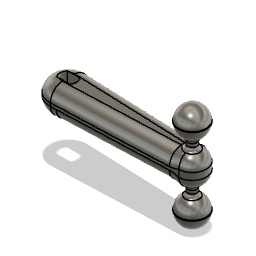
bicep (Autodesk Fusion 360 design; units mm, degrees)
Autodesk Fusion 360 part; units mm, degrees
sketch "Sketch1" plane through (0, 0, 0) normal (0, 1, 0) x (1, 0, 0)
  circle A0 centre (0, 0) radius 2.7
  line L0 (-2.056089, 1.75) -> (2.056089, 1.75)
  line L1 (-2.137171, -1.65) -> (2.137171, -1.65)
  circle A1 centre (0, 0) radius 6
  circle A2 centre (40, 0) radius 4.5
  line L2 (40.16875, 4.496835) -> (0.225, 5.99578)
  line L3 (0.225, -5.99578) -> (40.16875, -4.496835)
  circle A3 centre (40, 0) radius 1.5
  dimension "d1" = 5.4
  dimension "d2" = 3.4
  dimension "d3" = 1.75
  dimension "d4" = 12
  dimension "d10" = 9
  dimension "d11" = 40
  dimension "d14" = 3
  constraint coincident A0.centre A1.centre
  constraint horizontal L0
  constraint parallel L0 L1
  constraint concentric A0 A1
  constraint tangent A1 L2
  constraint tangent A2 L3
  constraint horizontal A0.centre A2.centre
  constraint tangent A1 L3
  constraint tangent A2 L2
  constraint concentric A2 A3
  measures "d1" diameter of A0
  measures "d2" distance of L0 L1
  measures "d3" distance of A0.centre L0
  measures "d4" diameter of A1
  measures "d10" diameter of A2
  measures "d11" distance of A0.centre A2.centre
  measures "d14" diameter of A3
extrude "Extrude1" add sketch "Sketch1" along normal blind 4.5 contours A0 L0 | A0 L1 | A1 | A1 A2 L2 L3 | A2 | A3 picked at (-0.377492, 2.168628) picked at (0.628341, -1.74435) picked at (-3.868944, -2.989429) picked at (15.82994, 0.496411) picked at (39.856155, 3.488694) picked at (39.627889, 0.265565)
extrude "Extrude2" add sketch "Sketch1" against normal blind 2.5 contours A0 L0 | A0 L1 | A1 | A1 A2 L2 L3 | A2 | A3 picked at (-0.377492, 2.168628) picked at (0.628341, -1.74435) picked at (-3.868944, -2.989429) picked at (15.82994, 0.496411) picked at (39.856155, 3.488694) picked at (39.627889, 0.265565)
sketch "Sketch2" plane through (0, 0, 0) normal (0, 1, 0) x (1, 0, 0)
extrude "Extrude3" add sketch "Sketch1" against normal blind 2 from surface at -2.5 contours A1 | A1 A2 L2 L3 | A2 | A3 picked at (-3.868944, -2.989429) picked at (15.82994, 0.496411) picked at (39.856155, 3.488694) picked at (39.627889, 0.265565)
extrude "Extrude4" add sketch "Sketch1" along normal mid plane 34 contours A3 picked at (39.627889, 0.265565)
extrude "Extrude5" add sketch "Sketch1" along normal blind 9 from surface at 8 contours A2 picked at (39.856155, 3.488694)
extrude "Extrude6" add sketch "Sketch1" against normal blind 9 from surface at -8 contours A2 picked at (39.856155, 3.488694)
fillet "Fillet1" radius 4.5 4 edges at (35.804527, -17, -1.627269) (35.804527, -8, 1.627269) (35.804527, 8, 1.627269) (35.804527, 17, 1.627269)
fillet "Fillet2" radius 1.5 1 edges at (38.601509, -4.5, 0.542423)
fillet "Fillet3" radius 1.5 1 edges at (38.601509, 4.5, -0.542423)
fillet "Fillet4" radius 1.5 2 edges at (38.601509, 8, -0.542423) (38.601509, -8, 0.542423)
fillet "Fillet5" radius 4 8 edges at (20.196875, -4.5, 5.246307) (-6, -4.5, 0) (20.196875, -4.5, -5.246307) (44.5, -4.5, 0) (20.196875, 4.5, 5.246307) (44.5, 4.5, 0) (20.196875, 4.5, -5.246307) (-6, 4.5, 0)
